Autodesk Inventor part; units mm, degrees
note: some values were not read from the file. Chosen so that the rebuilt part matches the saved one: direction of "Hole2".
(part 8 of 20)
  point P41 (-10089.727378, -10011.36586)
  point P42 (-10089.721398, -10011.390784)
  point P43 (-10089.71643, -10011.417432)
  point P44 (-10089.712492, -10011.445788)
  point P45 (-10089.709591, -10011.475889)
  point P46 (-10089.707712, -10011.507854)
  point P47 (-10089.706845, -10011.541631)
  point P48 (-10089.706982, -10011.577158)
  point P49 (-10089.708115, -10011.614374)
  point P50 (-10089.710236, -10011.653217)
  point P51 (-10091.342478, -10024.766723)
  point P52 (-10091.399992, -10024.634549)
  point P53 (-10091.454687, -10024.504325)
  point P54 (-10091.506613, -10024.375943)
  point P55 (-10091.602327, -10024.124275)
  point P56 (-10091.767293, -10025.369098)
  point P57 (-10091.726276, -10025.518742)
  point P58 (-10091.691392, -10025.662063)
  point P59 (-10091.66305, -10025.798056)
  point P60 (-10091.641632, -10025.925944)
  point P61 (-10091.627322, -10026.048439)
  point P62 (-10091.621155, -10026.162546)
  point P63 (-10091.621534, -10026.214773)
  point P64 (-10091.624365, -10026.263004)
  point P65 (-10091.629522, -10026.307033)
  point P66 (-10091.63684, -10026.346721)
  point P67 (-10091.646154, -10026.381929)
  point P68 (-10091.657297, -10026.412517)
  point P69 (-10091.685546, -10026.46165)
  point P70 (-10091.722424, -10026.49673)
  point P71 (-10091.767199, -10026.516512)
  point P72 (-10091.818874, -10026.520292)
  point P73 (-10091.875447, -10026.509788)
  point P74 (-10091.478055, -10022.118968)
  point P75 (-10091.547474, -10021.99281)
  point P76 (-10091.613916, -10021.868329)
  point P77 (-10091.67744, -10021.74542)
  point P78 (-10091.795946, -10021.503906)
  point P79 (-10091.795946, -10016.690075)
  point P80 (-10091.67744, -10016.448562)
  point P81 (-10091.613916, -10016.325653)
  point P82 (-10091.547474, -10016.201172)
  point P83 (-10091.478055, -10016.075014)
  point P84 (-10091.758883, -10022.729261)
  point P85 (-10091.707882, -10022.846777)
  point P86 (-10091.660376, -10022.960867)
  point P87 (-10091.616621, -10023.071034)
  point P88 (-10091.576871, -10023.176785)
  point P89 (-10091.541376, -10023.277639)
  point P90 (-10091.509756, -10023.375327)
  point P91 (-10091.482385, -10023.469454)
  point P92 (-10091.460347, -10023.557327)
  point P93 (-10091.444642, -10023.636373)
  point P94 (-10091.435434, -10023.705234)
  point P95 (-10091.432401, -10023.763266)
  point P96 (-10091.435236, -10023.810105)
  point P97 (-10091.443918, -10023.848166)
  point P98 (-10091.458396, -10023.877605)
  point P99 (-10091.458885, -10014.315907)
  point P100 (-10091.444621, -10014.344922)
  point P101 (-10091.435858, -10014.383099)
  point P102 (-10091.432679, -10014.430219)
  point P103 (-10091.435166, -10014.486064)
  point P104 (-10091.4434, -10014.550414)
  point P105 (-10091.457511, -10014.623566)
  point P106 (-10091.477418, -10014.705503)
  point P107 (-10091.502884, -10014.79549)
  point P108 (-10091.533671, -10014.89279)
  point P109 (-10091.56954, -10014.996669)
  point P110 (-10091.610254, -10015.106389)
  point P111 (-10091.655535, -10015.221179)
  point P112 (-10091.704831, -10015.339983)
  point P113 (-10091.602327, -10014.069706)
  point P114 (-10091.506613, -10013.818038)
  point P115 (-10091.454687, -10013.689656)
  point P116 (-10091.399992, -10013.559433)
  point P117 (-10091.342478, -10013.427258)
  point P118 (-10091.873857, -10011.683647)
  point P119 (-10091.817711, -10011.673522)
  point P120 (-10091.767253, -10011.677461)
  point P121 (-10091.723512, -10011.696704)
  point P122 (-10091.687035, -10011.731311)
  point P123 (-10091.658201, -10011.780891)
  point P124 (-10091.637389, -10011.845052)
  point P125 (-10091.624978, -10011.923403)
  point P126 (-10091.621158, -10012.016326)
  point P127 (-10091.625734, -10012.123495)
  point P128 (-10091.638501, -10012.243451)
  point P129 (-10091.659257, -10012.374739)
  point P130 (-10091.687797, -10012.5159)
  point P131 (-10091.723724, -10012.665293)
  point P132 (-10091.766103, -10012.820692)
  point P133 (-10070.533011, -10008.748999)
  point P134 (-10070.550101, -10008.752168)
  point P135 (-10070.56679, -10008.756332)
  point P136 (-10070.583016, -10008.761453)
  point P137 (-10070.598721, -10008.767492)
  point P138 (-10070.613843, -10008.774411)
  point P139 (-10070.628324, -10008.782172)
  point P140 (-10070.642102, -10008.790736)
  point P141 (-10070.655119, -10008.800064)
  point P142 (-10070.667313, -10008.81012)
  point P143 (-10070.678626, -10008.820863)
  point P144 (-10070.688996, -10008.832256)
  point P145 (-10070.698365, -10008.844261)
  point P146 (-10070.706672, -10008.856839)
  point P147 (-10070.713856, -10008.869951)
  point P148 (-10070.70671, -10009.029203)
  point P149 (-10070.699656, -10009.040668)
  point P150 (-10070.691833, -10009.051698)
  point P151 (-10070.683284, -10009.062271)
  point P152 (-10070.674052, -10009.072362)
  point P153 (-10070.664177, -10009.08195)
  point P154 (-10070.653702, -10009.091011)
  point P155 (-10070.64267, -10009.099522)
  point P156 (-10070.631122, -10009.107459)
  point P157 (-10070.6191, -10009.1148)
  point P158 (-10070.606647, -10009.121521)
  point P159 (-10070.593804, -10009.127599)
  point P160 (-10070.580613, -10009.133011)
  point P161 (-10070.567117, -10009.137734)
  point P162 (-10070.553358, -10009.141745)
  point P163 (-10070.560833, -10009.168396)
  point P164 (-10070.574308, -10009.163638)
  point P165 (-10070.587468, -10009.157958)
  point P166 (-10070.600283, -10009.151401)
  point P167 (-10070.612722, -10009.144012)
  point P168 (-10070.624756, -10009.135837)
  point P169 (-10070.636354, -10009.126921)
  point P170 (-10070.647488, -10009.11731)
  point P171 (-10070.658127, -10009.10705)
  point P172 (-10070.668242, -10009.096185)
  point P173 (-10070.677801, -10009.08476)
  point P174 (-10070.686776, -10009.072823)
  point P175 (-10070.695137, -10009.060417)
  point P176 (-10070.702854, -10009.047589)
  point P177 (-10070.709896, -10009.034384)
  point P178 (-10070.736958, -10008.893917)
  point P179 (-10070.733336, -10008.872545)
  point P180 (-10070.727426, -10008.851652)
  point P181 (-10070.719472, -10008.832002)
  point P182 (-10070.709661, -10008.813762)
  point P183 (-10070.698133, -10008.796927)
  point P184 (-10070.685027, -10008.781493)
  point P185 (-10070.670484, -10008.767455)
  point P186 (-10070.654642, -10008.754809)
  point P187 (-10070.63764, -10008.743551)
  point P188 (-10070.619619, -10008.733676)
  point P189 (-10070.600718, -10008.725181)
  point P190 (-10070.581076, -10008.71806)
  point P191 (-10070.560833, -10008.71231)
  point P192 (-10070.540128, -10008.707927)
  point P193 (-10070.388305, -10008.711852)
  point P194 (-10070.370582, -10008.717557)
  point P195 (-10070.353881, -10008.724776)
  point P196 (-10070.33824, -10008.733439)
  point P197 (-10070.323696, -10008.743478)
  point P198 (-10070.310287, -10008.754823)
  point P199 (-10070.29805, -10008.767405)
sketch "Sketch2" plane through (0, 0, 0) normal (1, 0, 0) x (0, 1, 0)
  line L0 (0, -156.78708) -> (0, 91.844197)
  line L1 (-13, 0) -> (12, 0)
  line L2 (-13, 0) -> (-13.762, 0)
  line L3 (-11, 25) -> (0, 25)
  line L4 (-11, 23.984) -> (-11, 25)
  line L5 (-8.5, 10) -> (8.5, 10)
  line L6 (8.5, 10) -> (8.5, 0)
  line L7 (8.5, 0) -> (-8.5, 0)
  line L8 (-8.5, 0) -> (-8.5, 10)
  line L9 (-12, 5) -> (12, 5)
  line L10 (12, 5) -> (12, 0)
  line L11 (12, 0) -> (-12, 0)
  line L12 (-12, 0) -> (-12, 5)
  line L13 (-7.484, 10) -> (-7.484, 0)
  line L14 (-10.984, 5) -> (-10.984, 0)
  spline S0 degree 4 poles (-11, 23.984) (-11, 20.713142) (-6.894492, 12.873224) (-7.998886, 10.368918) (-11.171855, 5.720689) (-13.556557, 3.508331) (-13.762, 1.387882) (-13.762, 0) knots 0 0 0 0 0 0.40323167 0.58584486 0.72553562 1 1 1 1 1
  spline S1 degree 4 poles (-10.457364, 23.213267) (-10.164256, 18.862838) (-2.980363, 8.550774) (-10.836637, 7.0695) (-13, 2.343966) (-13, 0) knots 0 0 0 0 0 0.54007932 1 1 1 1 1
  line L15 (-10.208157, 7.245893) -> (-13.791843, 2.754107) construction
  arc A0 (-10.476033, 6.706372) -> (-13.325291, 3.135118) centre (4.098236, -7.843675) ccw construction
  line L16 (-7.766531, 11.715278) -> (-9.233469, 8.284722) construction
  arc A1 (-9.226155, 8.730487) -> (-8.083773, 11.402041) centre (-14.334615, 12.494937) ccw construction
  line L17 (0, 23.984) -> (0, 25)
  line L18 (-13, 0) -> (-13, -15)
  line L19 (-13.762, 0) -> (-13.762, -15)
  arc A2 (-9.484, 23.984) -> (-10.457364, 23.213267) centre (-9.484, 22.984) ccw
  line L20 (-10.64831, 26.047373) -> (-10.266417, 20.379161) construction
  arc A3 (-10.271989, 25.399064) -> (-9.980462, 21.072091) centre (-3.224232, 23.700595) ccw construction
  line L21 (0, 23.984) -> (-9.484, 23.984)
  line L22 (-10.984, 23.984) -> (-11, 23.984)
  line L23 (-13.762, -15) -> (-13, -15)
  circle A4 centre (-10, 24) radius 1
  point P0 (0, 0)
  point P1 (0, 0)
  point P2 (0, 10)
  dimension "d16" = 25
  dimension "d17" = 17
  dimension "d18" = 10
  dimension "d19" = 24
  dimension "d20" = 5
  dimension "d22" = 1.016
  dimension "d23" = 1.016
  dimension "d25" = 2
  dimension "d26" = 15
  dimension "d27" = 0.762
  dimension "d28" = 13
  dimension "d91" = 11
  dimension "d92" = 2
  constraints: 46 end point, 10 parallel, 9 midpoint, 7 point on line, 5 centre point, 5 horizontal, 5 point on circle, 4 coincident, 4 perpendicular, 4 tangent, 3 vertical, 2 vertical alignment, 15 other
  measures "d16" distance between parallel lines of L1 L3
  measures "d17" distance between parallel lines of L6 L8
  measures "d18" distance between parallel lines of L7 L5
  measures "d19" distance between parallel lines of L10 L12
  measures "d20" distance between parallel lines of L11 L9
  measures "d22" distance between parallel lines of L13 L8
  measures "d23" distance between parallel lines of L14 L12
  measures "d25" diameter of A2
  measures "d26" distance of L19.end L2.end
  measures "d27" distance of L1.start L2.end
  measures "d28" distance of point (0, 0) L1.start
  measures "d91" distance of L3.end L3.start
  measures "d92" diameter of A4
revolve "Revolution1" [suppressed]
revolve "Mid Thick" add sketch "Sketch2" angle 360 about axis through (0, 0, -10) along (0, 0, 1) contours L2 L18 L23 L19
sketch "Sketch4" plane through (0, 0, 0) normal (1, 0, 0) x (0, 1, 0)
  line L0 (13.762, -15) -> (-13.762, -15)
  line L1 (0, -156.78708) -> (0, 91.844197)
  line L2 (-12, -15) -> (12, -15)
  line L3 (12, -15) -> (12, -29.976908)
  line L4 (12, -29.976908) -> (-12, -29.976908)
  line L5 (-12, -29.976908) -> (-12, -15)
  line L6 (-12, -29.976908) -> (-13.016, -29.976908)
  line L7 (-12, -25) -> (-12, -29.976908)
  line L8 (-13.762, -15) -> (-13.762, 0)
  line L9 (-13, 0) -> (-13, -15)
  spline S0 degree 4 poles (-13, -15) (-13, -16.878366) (-13, -20.635099) (-12, -24.341809) (-12, -28.098542) (-12, -29.976908) knots 0 0 0 0 0 0.5 1 1 1 1 1
  line L10 (-13.016, -29.976908) -> (-13.016, -27.488454)
  spline S1 degree 4 poles (-13.762, -15) (-13.762, -16.875595) (-13.762, -20.626785) (-13.016, -24.350123) (-13.016, -28.101313) (-13.016, -29.976908) knots 0 0 0 0 0 0.5 1 1 1 1 1
  line L11 (-13.762, -15) -> (-13, -15)
  point P0 (0, 0)
  point P1 (0, -15)
  point P2 (0, -15)
  dimension "d34" = 24
  dimension "d37" = 1.016
  constraints: 16 end point, 4 vertical, 3 parallel, 2 horizontal, 2 midpoint, 1 coincident, 1 collinear, 1 perpendicular, 1 point on line, 4 other
  measures "d34" distance between parallel lines of L3 L5
  measures "d37" distance of L4.end L6.end
revolve "Mid Tran" add sketch "Sketch4" angle 360 about axis through (0, 0, -10) along (0, 0, 1) contours S0 L6 S1 L0
sketch "Sketch5" plane through (0, 0, 0) normal (1, 0, 0) x (0, 1, 0)
  line L0 (13.016, -29.976908) -> (-13.016, -29.976908)
  line L1 (12, -29.976908) -> (-12, -29.976908)
  line L2 (0, -156.78708) -> (0, 91.844197)
  line L3 (-12, -29.976908) -> (14, -29.976908)
  line L4 (14, -29.976908) -> (14, -79.976908)
  line L5 (14, -79.976908) -> (-12, -79.976908)
  line L6 (-12, -79.976908) -> (-12, -29.976908)
  line L7 (-12, -29.976908) -> (-13.016, -29.976908)
  line L8 (-12, -79.976908) -> (-13.016, -79.976908)
  line L9 (-13.016, -79.976908) -> (-13.016, -29.976908)
  point P0 (0, 0)
  dimension "d39" = 26
  dimension "d40" = 1.016
  dimension "d41" = 50
  constraints: 14 end point, 3 parallel, 2 perpendicular, 1 horizontal
  measures "d39" distance between parallel lines of L4 L6
  measures "d40" distance of L5.end L8.end
  measures "d41" distance between parallel lines of L5 L0
revolve "Thin" add sketch "Sketch5" angle 360 about axis through (0, 0, -10) along (0, 0, 1) contours L6 L8 L9 L0
sketch "Sketch7" plane through (0, 0, -79.976908) normal (0, 0, -1) x (-1, 0, 0)
  circle A0 centre (0, 0) radius 13.016 projected
  circle A1 centre (0, 0) radius 12 projected
  circle A2 centre (0, 0) radius 13.016
  constraints: 1 centre point, 1 coincident, 1 concentric
ref_plane "Work Plane5" through (0, 0, -79.976908) normal (0, 0, 1) x (1, 0, 0)
extrude "Extrusion1" add sketch "Sketch7" along normal blind 4 contours A0 | A1
sketch "Sketch8" plane through (0, 0, -83.976908) normal (0, 0, -1) x (-1, 0, 0)
  circle A0 centre (0, 0) radius 13.016
  line L0 (7.582299, 2.074) -> (6.427599, 4.074)
  line L1 (6.427599, 4.074) -> (7.582299, 6.074)
  line L2 (7.582299, 6.074) -> (9.891701, 6.074)
  line L3 (9.891701, 6.074) -> (11.046401, 4.074)
  line L4 (11.046401, 4.074) -> (9.891701, 2.074)
  line L5 (9.891701, 2.074) -> (7.582299, 2.074)
  line L6 (0, -149.722214) -> (0, 130.927476)
  line L7 (-9.503701, 6.82) -> (-7.194299, 6.82)
  line L8 (-7.194299, 6.82) -> (-6.039599, 4.82)
  line L9 (-6.039599, 4.82) -> (-7.194299, 2.82)
  line L10 (-7.194299, 2.82) -> (-9.503701, 2.82)
  line L11 (-9.503701, 2.82) -> (-10.658401, 4.82)
  line L12 (-10.658401, 4.82) -> (-9.503701, 6.82)
  line L13 (1.154701, -7.494) -> (2.309401, -9.494)
  line L14 (2.309401, -9.494) -> (1.154701, -11.494)
  line L15 (1.154701, -11.494) -> (-1.154701, -11.494)
  line L16 (-1.154701, -11.494) -> (-2.309401, -9.494)
  line L17 (-2.309401, -9.494) -> (-1.154701, -7.494)
  line L18 (-1.154701, -7.494) -> (1.154701, -7.494)
  point P0 (8.737, 4.074)
  point P1 (-8.349, 4.82)
  point P2 (0, -9.494)
  point P3 (8.737, 4.074)
  dimension "d45" = 4.074
  dimension "d46" = 8.737
  dimension "d47" = 4.82
  dimension "d48" = 8.349
  dimension "d49" = 9.494
  dimension "d51" = 4
  dimension "d52" = 4
  dimension "d53" = 4
  constraints: 36 end point, 1 coincident, 1 other
  measures "d45" vertical distance of point (8.737, 4.074) A0.centre
  measures "d46" horizontal distance of point (8.737, 4.074) A0.centre
  measures "d47" vertical distance of point (-8.349, 4.82) A0.centre
  measures "d48" horizontal distance of A0.centre point (-8.349, 4.82)
  measures "d49" distance of point (0, -9.494) A0.centre
  measures "d51" distance between parallel lines of L0 L3
  measures "d52" distance between parallel lines of L7 L10
  measures "d53" distance between parallel lines of L13 L16
hole "Hole1" at (-8.737, 4.074, -83.976908) at (8.349, 4.82, -83.976908) at (0, -9.494, -83.976908) at (-8.737, 4.074, -83.976908) direction (0, 0, 1) diameter 1.778 depth 4 clearance for "Flat Head Machine Screw (82)" size "#0" standard "Ansi Unified Screw Threads"
sketch "Sketch9" plane through (0, 0, 0) normal (1, 0, 0) x (0, 1, 0)
  line L0 (-13.016, -83.976908) -> (-13.016, -29.976908)
  line L1 (13.016, -83.976908) -> (-13.016, -83.976908)
  line L2 (0, -156.78708) -> (0, 91.844197)
  line L3 (-8, -83.976908) -> (0, -83.976908)
  line L4 (0, -83.976908) -> (0, -103.976908)
  line L5 (0, -103.976908) -> (-5, -103.976908)
  spline S0 degree 3 poles (-13.016, -83.976908) (-13.016, -91.416878) (-13.016, -98.856848) (-5, -103.976908) knots 0 0 0 0 1 1 1 1
  line L6 (-13.016, -83.976908) -> (-8, -83.976908)
  point P0 (0, 0)
  point P1 (-4, -83.976908)
  dimension "d68" = 20
  dimension "d102" = 5
  constraints: 8 end point, 2 midpoint, 1 coincident, 1 horizontal, 1 horizontal alignment, 1 parallel, 1 perpendicular, 1 vertical, 2 other
  measures "d68" distance between parallel lines of L5 L3
  measures "d102" distance of L4.end L5.end
revolve "Revolution6" add sketch "Sketch9" angle 360 about axis through (0, 0, -10) along (0, 0, 1)
ref_plane "Work Plane6" through (0, 0, -82.476908) normal (0, 0, 1) x (1, 0, 0)
sketch "Sketch11" plane through (0, 0, -82.476908) normal (0, 0, 1) x (1, 0, 0)
  circle A0 centre (-8.737, 4.074) radius 0.889
  circle A1 centre (8.349, 4.82) radius 0.889
  circle A2 centre (0, -9.494) radius 0.889
  line L0 (-9.891701, 2.074) -> (-7.582299, 2.074)
  line L1 (-11.046401, 4.074) -> (-9.891701, 2.074)
  line L2 (-7.582299, 2.074) -> (-6.427599, 4.074)
  line L3 (-9.891701, 6.074) -> (-11.046401, 4.074)
  line L4 (-7.582299, 6.074) -> (-9.891701, 6.074)
  line L5 (-6.427599, 4.074) -> (-7.582299, 6.074)
  line L6 (1.154701, -7.494) -> (-1.154701, -7.494)
  line L7 (2.309401, -9.494) -> (1.154701, -7.494)
  line L8 (1.154701, -11.494) -> (2.309401, -9.494)
  line L9 (-1.154701, -11.494) -> (1.154701, -11.494)
  line L10 (-2.309401, -9.494) -> (-1.154701, -11.494)
  line L11 (-1.154701, -7.494) -> (-2.309401, -9.494)
  line L12 (7.194299, 6.82) -> (6.039599, 4.82)
  line L13 (9.503701, 6.82) -> (7.194299, 6.82)
  line L14 (10.658401, 4.82) -> (9.503701, 6.82)
  line L15 (9.503701, 2.82) -> (10.658401, 4.82)
  line L16 (7.194299, 2.82) -> (9.503701, 2.82)
  line L17 (6.039599, 4.82) -> (7.194299, 2.82)
  point P0 (0, 0)
extrude "Extrusion3" cut sketch "Sketch11" against normal through all contours A0 | A1 | A2 | L1 L3 L4 L5 L2 L0 | L7 L8 L9 L10 L11 L6 | L13 L14 L15 L16 L17 L12
ref_plane "Work Plane7" through (0, 0, -79.976908) normal (0, 0, 1) x (1, 0, 0)
hole "Hole2" at (0, 0, -103.976908) direction (0, 0, 1) diameter 10 depth 24
sketch "Sketch12" plane through (0, 0, 0) normal (1, 0, 0) x (0, 1, 0)
  spline S0 degree 3 poles (67.040686, -110.340683) (67.181711, -110.754373) (67.468131, -111.594574) (67.844542, -112.900649) (68.165475, -114.276843) (68.403591, -115.689425) (68.553461, -117.090576) (68.628909, -118.438876) (68.654169, -119.741368) (68.654209, -120.596035) (68.654229, -121.018326) knots 0 0 0 0 0.13110718 0.26627767 0.40758133 0.55482273 0.69573025 0.83010398 0.95981582 1.08650249 1.08650249 1.08650249 1.08650249
  spline S1 degree 3 poles (65.040686, -106.036195) (65.040686, -106.035984) (65.040686, -106.035137) (65.040686, -106.033234) (65.040686, -106.030066) (65.040686, -106.025636) (65.040686, -106.019951) (65.040686, -106.013017) (65.040686, -106.004838) (65.040686, -105.99542) (65.040686, -105.984769) (65.040686, -105.972891) (65.040686, -105.959801) (65.040686, -105.945517) (65.040686, -105.930056) (65.040686, -105.913432) (65.040686, -105.895658) (65.040686, -105.883426) (65.040686, -105.877121) knots 0 0 0 0 0.00398745 0.01595749 0.03589091 0.06374884 0.09949715 0.14310174 0.1945285 0.2537433 0.32071204 0.39540061 0.47774624 0.56757484 0.66479437 0.76932497 0.8810868 1 1 1 1
  spline S2 degree 3 poles (65.040686, -105.877121) (65.194176, -106.260743) (65.498781, -107.022054) (66.173784, -108.506895) (66.69415, -109.607645) (67.040686, -110.340683) knots 0 0 0 0 0.25334256 0.50276707 1 1 1 1
  spline S3 degree 3 poles (83.354686, -109.977444) (83.205067, -110.403955) (82.900857, -111.271152) (82.494774, -112.619657) (82.145236, -114.043985) (81.88387, -115.507795) (81.718837, -116.959462) (81.635693, -118.354075) (81.607874, -119.699651) (81.607833, -120.582214) (81.607812, -121.018326) knots 0 0 0 0 0.13558682 0.27568002 0.42231514 0.57532331 0.7214304 0.86036495 0.99429907 1.12513191 1.12513191 1.12513191 1.12513191
  line L0 (81.354686, -105.464425) -> (81.354686, -121.018326)
  line L1 (81.607812, -121.018326) -> (81.354686, -121.018326)
  line L2 (81.354686, -121.018326) -> (79.354686, -121.018326)
  spline S4 degree 3 poles (79.354686, -121.018326) (79.354686, -120.136015) (79.354686, -118.791551) (79.354686, -116.963337) (79.354686, -115.515321) (79.354686, -114.054436) (79.354686, -112.629922) (79.354686, -111.279853) (79.354686, -110.404808) (79.354686, -109.977141) knots 0 0 0 0 0.26469338 0.4033392 0.54846434 0.69909791 0.84160494 0.97581833 1.10411856 1.10411856 1.10411856 1.10411856
  spline S5 degree 3 poles (79.354686, -109.977141) (79.707447, -109.240902) (80.237826, -108.133962) (80.818531, -106.821015) (81.133082, -106.053241) (81.280528, -105.661469) (81.354686, -105.464425) knots 0 0 0 0 0.49596798 0.74569065 0.8720938 1 1 1 1
  spline S6 degree 3 poles (81.354686, -105.464425) (81.436258, -105.489435) (81.598942, -105.539315) (81.848975, -105.589935) (82.101098, -105.62152) (82.354754, -105.631933) (82.608329, -105.621551) (82.860555, -105.589985) (83.110519, -105.539404) (83.273215, -105.489542) (83.354686, -105.464572) knots 0 0 0 0 0.12572609 0.25074567 0.37552827 0.50000542 0.62458391 0.74924522 0.87443269 1 1 1 1
  spline S7 degree 3 poles (83.354686, -105.464572) (83.354686, -105.853913) (83.354686, -106.619619) (83.354686, -108.123909) (83.354686, -109.238859) (83.354686, -109.977444) knots 0 0 0 0 0.25882001 0.5090148 1 1 1 1
  line L3 (67.040686, -94.518326) -> (67.040686, -110.340683)
  line L4 (67.040686, -94.518326) -> (69.040686, -94.518326)
  line L5 (69.040686, -94.518326) -> (69.040686, -121.018326)
  line L6 (65.040686, -94.518326) -> (65.040686, -105.877121)
  line L7 (65.040686, -94.518326) -> (67.040686, -94.518326)
  line L8 (79.354686, -94.518326) -> (79.354686, -109.977141)
  line L9 (79.354686, -94.518326) -> (81.354686, -94.518326)
  line L10 (81.354686, -94.518326) -> (81.354686, -105.464425)
  line L11 (81.354686, -94.518326) -> (83.354686, -94.518326)
  line L12 (83.354686, -94.518326) -> (83.354686, -105.464572)
  line L13 (78.608686, -94.518326) -> (78.608686, -121.018326)
  line L14 (78.608686, -94.518326) -> (79.354686, -94.518326)
  line L15 (80.608686, -94.518326) -> (80.608686, -121.018326)
  line L16 (82.608686, -94.518326) -> (82.608686, -110.485254)
  spline S8 degree 3 poles (80.987443, -121.018326) (80.987462, -120.601747) (80.987501, -119.758823) (81.01289, -118.474335) (81.088746, -117.144746) (81.239448, -115.762632) (81.478869, -114.368665) (81.801344, -113.01032) (82.179342, -111.721556) (82.467066, -110.89305) (82.608686, -110.485254) knots 0 0 0 0 0.12497306 0.25287553 0.38537145 0.52436553 0.66974205 0.80937847 0.9429718 1.07246485 1.07246485 1.07246485 1.07246485
  spline S9 degree 3 poles (82.608686, -105.721075) (82.52253, -105.726584) (82.350319, -105.737597) (82.091245, -105.726689) (81.83373, -105.695808) (81.578795, -105.643474) (81.327626, -105.571102) (81.081461, -105.479205) (80.840427, -105.370299) (80.686114, -105.284214) (80.608686, -105.24102) knots 0 0 0 0 0.12386032 0.2475762 0.37158497 0.495852 0.6207493 0.74643209 0.87276965 1 1 1 1
  spline S10 degree 3 poles (80.608686, -105.24102) (80.536619, -105.426978) (80.393173, -105.797117) (80.085372, -106.522873) (79.67593, -107.411332) (79.152243, -108.458702) (78.790042, -109.149046) (78.608686, -109.494703) knots 0 0 0 0 0.12719878 0.25318248 0.50275428 0.75102731 1 1 1 1
  line L17 (88.534686, -92.018326) -> (64.534686, -92.018326)
  line L18 (86.018686, 21.942582) -> (67.050686, 21.942582)
  line L19 (86.505368, 21.557215) -> (66.564004, 21.557215)
  spline S11 degree 3 poles (65.550686, 2.958582) (65.696442, 3.15771) (65.990398, 3.559307) (66.63789, 4.332671) (67.316977, 5.091944) (67.96316, 5.888495) (68.33248, 6.417332) (68.593779, 6.863991) (68.769836, 7.213831) (68.926202, 7.578332) (69.008957, 7.831116) (69.050686, 7.958582) knots 0 0 0 0 0.07401284 0.14926686 0.30244691 0.37959616 0.45685507 0.49566205 0.53474567 0.5742877 0.61450742 0.61450742 0.61450742 0.61450742
  spline S12 degree 3 poles (87.518686, 2.958582) (87.37293, 3.15771) (87.078974, 3.559307) (86.431482, 4.332671) (85.752395, 5.091944) (85.106213, 5.888495) (84.736892, 6.417332) (84.475593, 6.863991) (84.299536, 7.213831) (84.14317, 7.578332) (84.060415, 7.831116) (84.018686, 7.958582) knots 0 0 0 0 0.07401284 0.14926686 0.30244691 0.37959616 0.45685507 0.49566205 0.53474567 0.5742877 0.61450742 0.61450742 0.61450742 0.61450742
  spline S13 degree 3 poles (64.034686, -2.041418) (64.037832, -1.818607) (64.04412, -1.373262) (64.103581, -0.708699) (64.209137, -0.052784) (64.368677, 0.589154) (64.583246, 1.213523) (64.853982, 1.817393) (65.174985, 2.402355) (65.424915, 2.772377) (65.550686, 2.958582) knots 0 0 0 0 0.06683217 0.13358148 0.19996019 0.26595386 0.33177154 0.39774949 0.46426825 0.53165054 0.53165054 0.53165054 0.53165054
  spline S14 degree 3 poles (89.034686, -2.041418) (89.03154, -1.818607) (89.025252, -1.373262) (88.965791, -0.708699) (88.860235, -0.052784) (88.700695, 0.589154) (88.486126, 1.213523) (88.215391, 1.817393) (87.894387, 2.402355) (87.644457, 2.772377) (87.518686, 2.958582) knots 0 0 0 0 0.06683217 0.13358148 0.19996019 0.26595386 0.33177154 0.39774949 0.46426825 0.53165054 0.53165054 0.53165054 0.53165054
  arc A0 (86.505368, 21.557215) -> (86.018686, 21.942582) centre (86.018686, 21.442582) ccw
  arc A1 (67.050686, 21.942582) -> (66.564004, 21.557215) centre (67.050686, 21.442582) ccw
  spline S15 degree 3 poles (69.050686, 7.958582) (69.104819, 8.159433) (69.215638, 8.570605) (69.299992, 9.222432) (69.32743, 9.914929) (69.289863, 10.650133) (69.193528, 11.426673) (69.041848, 12.243358) (68.83889, 13.097233) (68.505279, 14.303469) (68.009186, 15.861647) (67.384973, 17.757913) (66.925594, 19.360458) (66.657385, 20.629559) (66.594637, 21.25291) (66.564004, 21.557215) knots 0 0 0 0 0.06234657 0.1276327 0.1966407 0.27004939 0.34820305 0.43123424 0.51911498 0.61142292 0.80662861 1.00959387 1.21035176 1.30648489 1.39817641 1.39817641 1.39817641 1.39817641
  spline S16 degree 3 poles (84.018686, 7.958582) (83.964553, 8.159433) (83.853734, 8.570605) (83.769381, 9.222432) (83.741942, 9.914929) (83.77951, 10.650133) (83.875844, 11.426673) (84.027524, 12.243358) (84.230482, 13.097233) (84.564093, 14.303469) (85.060187, 15.861647) (85.684399, 17.757913) (86.143778, 19.360458) (86.411987, 20.629559) (86.474736, 21.25291) (86.505368, 21.557215) knots 0 0 0 0 0.06234657 0.1276327 0.1966407 0.27004939 0.34820305 0.43123424 0.51911498 0.61142292 0.80662861 1.00959387 1.21035176 1.30648489 1.39817641 1.39817641 1.39817641 1.39817641
  line L20 (87.534686, 22.958582) -> (65.534686, 22.958582)
  spline S17 degree 3 poles (68.034686, 7.958582) (67.934145, 7.742514) (67.730909, 7.305746) (67.355975, 6.67586) (66.947859, 6.044593) (66.506986, 5.411639) (66.037254, 4.782076) (65.376039, 3.96496) (64.87044, 3.36019) (64.534686, 2.958582) knots 0 0 0 0 0.07145122 0.1444341 0.21963753 0.29697342 0.37578786 0.45523025 0.61227239 0.61227239 0.61227239 0.61227239
  spline S18 degree 3 poles (85.034686, 7.958582) (85.135227, 7.742514) (85.338463, 7.305746) (85.713398, 6.67586) (86.121513, 6.044593) (86.562387, 5.411639) (87.032119, 4.782076) (87.693333, 3.96496) (88.198933, 3.36019) (88.534686, 2.958582) knots 0 0 0 0 0.07145122 0.1444341 0.21963753 0.29697342 0.37578786 0.45523025 0.61227239 0.61227239 0.61227239 0.61227239
  spline S19 degree 3 poles (64.534686, 2.958582) (64.391139, 2.773942) (64.177438, 2.499066) (63.921801, 2.115667) (63.74796, 1.825722) (63.592502, 1.530213) (63.456028, 1.22896) (63.339682, 0.921485) (63.243369, 0.607961) (63.166118, 0.288773) (63.087618, -0.145209) (63.032036, -0.699119) (63.015615, -1.369168) (63.017663, -1.817428) (63.018686, -2.041418) knots 0 0 0 0 0.07013118 0.1044054 0.13817293 0.17150982 0.2045203 0.23732848 0.27006639 0.30285264 0.33579 0.40230943 0.46959172 0.53678969 0.53678969 0.53678969 0.53678969
  spline S20 degree 3 poles (88.534686, 2.958582) (88.678233, 2.773942) (88.891934, 2.499066) (89.147571, 2.115667) (89.321413, 1.825722) (89.476871, 1.530213) (89.613344, 1.22896) (89.72969, 0.921485) (89.826003, 0.607961) (89.903254, 0.288773) (89.981754, -0.145209) (90.037337, -0.699119) (90.053758, -1.369168) (90.05171, -1.817428) (90.050686, -2.041418) knots 0 0 0 0 0.07013118 0.1044054 0.13817293 0.17150982 0.2045203 0.23732848 0.27006639 0.30285264 0.33579 0.40230943 0.46959172 0.53678969 0.53678969 0.53678969 0.53678969
  spline S21 degree 3 poles (65.534686, 21.942582) (65.55153, 21.625542) (65.586982, 20.958222) (65.799755, 19.936612) (66.079405, 18.863014) (66.530055, 17.400852) (67.022889, 15.959413) (67.492662, 14.551628) (67.805168, 13.564577) (68.06678, 12.638691) (68.268386, 11.780568) (68.404564, 10.992675) (68.468083, 10.273449) (68.458204, 9.618811) (68.379378, 9.021526) (68.239024, 8.4702) (68.102158, 8.127516) (68.034686, 7.958582) knots 0 0 0 0 0.09512154 0.200216 0.31218274 0.42803367 0.65906444 0.76919754 0.87325746 0.96964043 1.05776849 1.13759246 1.20931346 1.27406394 1.33359113 1.38967504 1.44420495 1.44420495 1.44420495 1.44420495
  spline S22 degree 3 poles (87.534686, 21.942582) (87.517843, 21.625542) (87.48239, 20.958222) (87.269617, 19.936612) (86.989967, 18.863014) (86.539318, 17.400852) (86.046483, 15.959413) (85.57671, 14.551628) (85.264205, 13.564577) (85.002592, 12.638691) (84.800986, 11.780568) (84.664809, 10.992675) (84.60129, 10.273449) (84.611168, 9.618811) (84.689994, 9.021526) (84.830348, 8.4702) (84.967214, 8.127516) (85.034686, 7.958582) knots 0 0 0 0 0.09512154 0.200216 0.31218274 0.42803367 0.65906444 0.76919754 0.87325746 0.96964043 1.05776849 1.13759246 1.20931346 1.27406394 1.33359113 1.38967504 1.44420495 1.44420495 1.44420495 1.44420495
  line L21 (65.534686, 21.942582) -> (65.534686, 22.958582)
  line L22 (87.534686, 21.942582) -> (87.534686, 22.958582)
  line L23 (84.534686, -121.018326) -> (81.607812, -121.018326)
  line L24 (79.354686, -121.018326) -> (68.654229, -121.018326)
  spline S23 degree 3 poles (63.518686, -96.018326) (63.519479, -96.870586) (63.520667, -98.146747) (63.621473, -99.842752) (63.759935, -101.104322) (63.970024, -102.355857) (64.256379, -103.595658) (64.611615, -104.825029) (64.897293, -105.631431) (65.040686, -106.036195) knots 0 0 0 0 0.25561003 0.38274706 0.50949551 0.6361782 0.76322409 0.89103186 1.01983443 1.01983443 1.01983443 1.01983443
  spline S24 degree 3 poles (89.550686, -96.018326) (89.546142, -97.088345) (89.539339, -98.690067) (89.355839, -100.815549) (89.097312, -102.390762) (88.720342, -103.947002) (88.078134, -106.008624) (87.042686, -108.518326) (86.007238, -111.028028) (85.36503, -113.08965) (84.98806, -114.645891) (84.729533, -116.221103) (84.546034, -118.346586) (84.539231, -119.948307) (84.534686, -121.018326) knots 0 0 0 0 0.32084871 0.48028147 0.63946219 0.79924314 0.96029185 1.28673686 1.61318187 1.77423059 1.93401153 2.09319225 2.25262502 2.57347372 2.57347372 2.57347372 2.57347372
  line L25 (81.534686, -92.018326) -> (81.534686, -121.018326)
  line L26 (71.534686, -92.018326) -> (71.534686, -121.018326)
  line L27 (81.497686, -92.018326) -> (81.497686, -94.518326)
  line L28 (79.719686, -92.018326) -> (79.719686, -94.518326)
  line L29 (82.243686, -92.018326) -> (82.243686, -94.518326)
  line L30 (80.465686, -92.018326) -> (80.465686, -94.518326)
  line L31 (67.929686, -92.018326) -> (67.929686, -94.518326)
  line L32 (66.151686, -92.018326) -> (66.151686, -94.518326)
  line L33 (64.534686, -92.018326) -> (64.534686, -32.018326)
  line L34 (88.534686, -92.018326) -> (88.534686, -32.018326)
  line L35 (63.518686, -96.018326) -> (63.518686, -32.018326)
  line L36 (89.550686, -96.018326) -> (89.550686, -32.018326)
  spline S25 degree 3 poles (64.534686, -32.018326) (64.534349, -31.809534) (64.533674, -31.392358) (64.495675, -30.767061) (64.408772, -30.145712) (64.284686, -29.529872) (64.1606, -28.914033) (64.073697, -28.292684) (64.035698, -27.667387) (64.035024, -27.250211) (64.034686, -27.041418) knots 0 0 0 0 0.0626312 0.12513986 0.18776052 0.25067229 0.31358405 0.37620471 0.43871337 0.50134457 0.50134457 0.50134457 0.50134457
  spline S26 degree 3 poles (88.534686, -32.018326) (88.535024, -31.809534) (88.535698, -31.392358) (88.573697, -30.767061) (88.6606, -30.145712) (88.784686, -29.529872) (88.908772, -28.914033) (88.995675, -28.292684) (89.033674, -27.667387) (89.034349, -27.250211) (89.034686, -27.041418) knots 0 0 0 0 0.0626312 0.12513986 0.18776052 0.25067229 0.31358405 0.37620471 0.43871337 0.50134457 0.50134457 0.50134457 0.50134457
  spline S27 degree 3 poles (63.018686, -27.041418) (63.019024, -27.250211) (63.019698, -27.667387) (63.057697, -28.292684) (63.1446, -28.914033) (63.268686, -29.529872) (63.392772, -30.145712) (63.479675, -30.767061) (63.517674, -31.392358) (63.518349, -31.809534) (63.518686, -32.018326) knots 0 0 0 0 0.0626312 0.12513986 0.18776052 0.25067229 0.31358405 0.37620471 0.43871337 0.50134457 0.50134457 0.50134457 0.50134457
  spline S28 degree 3 poles (90.050686, -27.041418) (90.050349, -27.250211) (90.049674, -27.667387) (90.011675, -28.292684) (89.924772, -28.914033) (89.800686, -29.529872) (89.6766, -30.145712) (89.589697, -30.767061) (89.551698, -31.392358) (89.551024, -31.809534) (89.550686, -32.018326) knots 0 0 0 0 0.0626312 0.12513986 0.18776052 0.25067229 0.31358405 0.37620471 0.43871337 0.50134457 0.50134457 0.50134457 0.50134457
  line L37 (64.034686, -27.041418) -> (64.034686, -2.041418)
  line L38 (89.034686, -27.041418) -> (89.034686, -2.041418)
  line L39 (63.018686, -27.041418) -> (63.018686, -2.041418)
  line L40 (90.050686, -27.041418) -> (90.050686, -2.041418)
  line L41 (-90.466621, -35.917041) -> (-90.442087, -35.912003)
  ellipse E0 centre (-90.343602, -35.894235) end of major axis (-89.559894, -35.733604) minor radius 0.002388 (-90.187105, -35.859771) -> (-90.442087, -35.912003) ccw
  ellipse E1 centre (-90.343602, -35.894235) end of major axis (-89.559894, -35.733604) minor radius 0.002388 (-89.559894, -35.733604) -> (-90.01196, -35.824053) ccw
  line L42 (-89.559756, -35.73428) -> (-89.559894, -35.733604)
  ellipse E2 centre (-103.65948, -35.894235) end of major axis (-104.443188, -35.733604) minor radius 0.002388 (-103.992479, -35.823777) -> (-104.443188, -35.733604) ccw
  line L43 (-102.646483, -36.098913) -> (-102.414014, -36.146449)
  line L44 (-104.443326, -35.73428) -> (-104.443188, -35.733604)
  ellipse E3 centre (-90.875964, -36.03792) end of major axis (-90.117864, -35.782412) minor radius 0.00228 (-90.80754, -36.012462) -> (-90.958968, -36.063503) ccw
  ellipse E4 centre (-90.875964, -36.03792) end of major axis (-90.117864, -35.782412) minor radius 0.00228 (-90.689307, -35.972678) -> (-90.801699, -36.010495) ccw
  ellipse E5 centre (-90.875964, -36.03792) end of major axis (-90.117864, -35.782412) minor radius 0.00228 (-90.117864, -35.782412) -> (-90.289361, -35.838691) ccw
  line L45 (-90.11513, -35.790524) -> (-90.117864, -35.782412)
  line L46 (-92.674489, -35.892021) -> (-94.327933, -30.986199)
  ellipse E6 centre (-88.233607, -36.951348) end of major axis (-89.011017, -37.140116) minor radius 0.136933 (-88.528399, -36.890417) -> (-88.545422, -36.895726) ccw
  line L47 (-88.816146, -36.96257) -> (-88.62556, -36.912263)
  ellipse E7 centre (-88.00113, -37.90877) end of major axis (-88.487012, -38.02675) minor radius 0.085583 (-88.121508, -37.851839) -> (-88.268041, -38.045128) ccw
  ellipse E8 centre (-106.692039, -35.867548) end of major axis (-107.491785, -35.8877) minor radius 0.133925 (-107.04331, -35.755799) -> (-107.491785, -35.8877) ccw
  line L48 (-106.719125, -35.734323) -> (-105.145649, -35.686856)
  line L49 (-105.145649, -35.686856) -> (-105.140676, -35.88423)
  ellipse E9 centre (-106.642372, -37.838699) end of major axis (-107.442118, -37.85885) minor radius 0.133925 (-106.370354, -37.706058) -> (-106.669458, -37.705473) ccw
  line L50 (-105.145649, -35.686856) -> (-105.155563, -35.29341)
  line L51 (-105.172568, -34.618497) -> (-105.1969, -33.652856)
  ellipse E10 centre (-107.037224, -22.168053) end of major axis (-109.126561, -22.220698) minor radius 0.349879 (-107.891271, -21.869557) -> (-108.146045, -21.898574) ccw
  ellipse E11 centre (-107.014874, -23.055071) end of major axis (-109.104211, -23.107715) minor radius 0.349879 (-107.877588, -22.757441) -> (-108.11313, -22.784232) ccw
  ellipse E12 centre (-107.014874, -23.055071) end of major axis (-108.514398, -23.092854) minor radius 0.251109 (-106.221205, -22.822514) -> (-108.470628, -23.150977) ccw
  ellipse E13 centre (-106.642372, -37.838699) end of major axis (-107.142214, -37.851293) minor radius 0.083703 (-106.716086, -37.757691) -> (-106.890842, -37.917435) ccw
  ellipse E14 centre (-104.240205, -35.814279) end of major axis (-105.038162, -35.757144) minor radius 0.002347 (-104.354333, -35.803779) -> (-105.038162, -35.757144) ccw
  line L52 (-104.354333, -35.803779) -> (-104.295665, -35.807955)
  line L53 (-104.059089, -35.824793) -> (-102.799639, -35.914435)
  line L54 (-102.799639, -35.914435) -> (-102.814933, -36.128042)
  line L55 (-105.039107, -35.770331) -> (-105.038162, -35.757144)
  line L56 (-102.799639, -35.914435) -> (-102.680421, -34.24943)
  line L57 (-90.880231, -35.479301) -> (-90.812485, -35.821466)
  line L58 (-91.848425, -36.30283) -> (-90.375139, -36.031417)
  ellipse E15 centre (-90.307773, -35.920377) end of major axis (-89.523007, -35.765) minor radius 0.096422 (-90.375139, -36.031417) -> (-89.66586, -35.73864) ccw
  line L59 (-89.66586, -35.73864) -> (-90.18766, -35.747597)
  line L60 (-89.521474, -35.772742) -> (-89.523007, -35.765)
  line L61 (-88.366054, -35.597257) -> (-88.355181, -35.701091)
  line L62 (-88.871729, -35.904988) -> (-87.996085, -35.808354)
  ellipse E16 centre (-87.889599, -35.831286) end of major axis (-87.093949, -35.747968) minor radius 0.034185 (-87.129232, -35.741687) -> (-87.996085, -35.808354) ccw
  ellipse E17 centre (-89.335927, -22.019504) end of major axis (-87.257293, -21.801836) minor radius 0.089309 (-87.399609, -21.784456) -> (-87.900814, -21.804539) ccw
  ellipse E18 centre (-89.24228, -22.913792) end of major axis (-87.163646, -22.696124) minor radius 0.089309 (-87.308637, -22.678729) -> (-87.376049, -22.679181) ccw
  ellipse E19 centre (-87.681494, -37.818593) end of major axis (-88.178775, -37.870667) minor radius 0.021366 (-88.057958, -37.843906) -> (-88.155364, -37.861609) ccw
  ellipse E20 centre (-87.681494, -37.818593) end of major axis (-87.184213, -37.766519) minor radius 0.021366 (-87.224132, -37.762354) -> (-87.493652, -37.779068) ccw
  ellipse E21 centre (-100.301556, -37.154438) end of major axis (-99.595388, -37.300356) minor radius 0.431228 (-101.009802, -37.10384) -> (-100.993099, -37.166903) ccw
  line L63 (-104.697671, -35.209096) -> (-104.756287, -35.768848)
  ellipse E22 centre (-106.113483, -35.831286) end of major axis (-105.317834, -35.914604) minor radius 0.034185 (-106.14405, -35.793745) -> (-106.846869, -35.7413) ccw
  line L64 (-106.14405, -35.793745) -> (-105.130983, -35.897952)
  line L65 (-104.561105, -35.784903) -> (-104.501911, -35.219625)
  ellipse E23 centre (-104.667155, -22.019504) end of major axis (-106.745789, -21.801836) minor radius 0.089309 (-106.102268, -21.804539) -> (-106.603473, -21.784456) ccw
  ellipse E24 centre (-104.760802, -22.913792) end of major axis (-106.839436, -22.696124) minor radius 0.089309 (-106.627033, -22.679181) -> (-106.694445, -22.678729) ccw
  ellipse E25 centre (-104.760802, -22.913792) end of major axis (-106.252645, -22.757571) minor radius 0.064098 (-106.212405, -22.747195) -> (-106.215765, -22.775958) ccw
  ellipse E26 centre (-106.321588, -37.818593) end of major axis (-105.824307, -37.870667) minor radius 0.021366 (-105.855185, -37.874796) -> (-105.945124, -37.843906) ccw
  ellipse E27 centre (-106.321588, -37.818593) end of major axis (-106.818869, -37.766519) minor radius 0.021366 (-106.50943, -37.779068) -> (-106.787599, -37.777382) ccw
  line L66 (-101.826025, -33.176696) -> (-102.425721, -36.205579)
  line L67 (-104.130028, -35.752776) -> (-104.207956, -35.745992)
  ellipse E28 centre (-103.695309, -35.920377) end of major axis (-104.480075, -35.765) minor radius 0.096422 (-104.207956, -35.745992) -> (-103.820309, -35.993013) ccw
  line L68 (-103.820309, -35.993013) -> (-102.294711, -36.321317)
  line L69 (-102.294711, -36.321317) -> (-102.303894, -36.367694)
  line L70 (-104.481608, -35.772742) -> (-104.480075, -35.765)
  line L71 (-102.350104, -36.286019) -> (-102.294711, -36.321317)
  line L72 (-102.294711, -36.321317) -> (-101.67558, -33.194274)
  line L73 (-90.012444, -35.829859) -> (-89.844365, -35.817773)
  ellipse E29 centre (-89.762877, -35.814279) end of major axis (-88.96492, -35.757144) minor radius 0.002347 (-88.96492, -35.757144) -> (-89.844365, -35.817773) ccw
  line L74 (-88.963976, -35.770331) -> (-88.96492, -35.757144)
  line L75 (-91.608122, -33.121203) -> (-91.608901, -33.110315)
  line L76 (-87.734507, -35.527633) -> (-87.739358, -35.720134)
  line L77 (-88.95241, -35.73049) -> (-87.421684, -35.732161)
  ellipse E30 centre (-87.311043, -35.867548) end of major axis (-86.511297, -35.8877) minor radius 0.133925 (-86.511297, -35.8877) -> (-87.421684, -35.732161) ccw
  ellipse E31 centre (-86.965858, -22.168053) end of major axis (-89.055195, -22.115408) minor radius 0.349879 (-85.857037, -21.898574) -> (-86.111811, -21.869557) ccw
  ellipse E32 centre (-86.988208, -23.055071) end of major axis (-89.077545, -23.002426) minor radius 0.349879 (-85.889952, -22.784232) -> (-86.125494, -22.757441) ccw
  ellipse E33 centre (-86.988208, -23.055071) end of major axis (-85.488684, -23.092854) minor radius 0.251109 (-85.552513, -23.162744) -> (-87.781877, -22.822514) ccw
  ellipse E34 centre (-87.335876, -36.853124) end of major axis (-88.135623, -36.832973) minor radius 0.133925 (-87.446517, -36.717736) -> (-87.466538, -36.717758) ccw
  ellipse E35 centre (-87.36071, -37.838699) end of major axis (-87.860551, -37.826104) minor radius 0.083703 (-87.11224, -37.917435) -> (-87.089062, -37.915636) ccw
  ellipse E36 centre (-87.36071, -37.838699) end of major axis (-86.860869, -37.851293) minor radius 0.083703 (-87.035815, -37.783027) -> (-87.286996, -37.757691) ccw
  line L78 (-105.300401, -36.919594) -> (-105.186074, -36.946173)
  ellipse E37 centre (-105.769475, -36.951348) end of major axis (-106.546885, -36.762581) minor radius 0.136933 (-105.45766, -36.895726) -> (-105.476237, -36.889936) ccw
  ellipse E38 centre (-106.001952, -37.90877) end of major axis (-105.516071, -38.02675) minor radius 0.085583 (-105.735041, -38.045128) -> (-105.881574, -37.851839) ccw
  ellipse E39 centre (-103.127118, -36.03792) end of major axis (-103.885218, -35.782412) minor radius 0.00228 (-103.715025, -35.838256) -> (-103.885218, -35.782412) ccw
  line L79 (-101.907552, -36.988982) -> (-102.062587, -37.448979)
  line L80 (-103.887952, -35.790524) -> (-103.885218, -35.782412)
  line L81 (-101.002593, -34.303939) -> (-99.76883, -30.643326)
  line L82 (-101.823309, -37.323227) -> (-102.062587, -37.448979)
  line L83 (-102.062587, -37.448979) -> (-102.085947, -37.441338)
  line L84 (-102.385663, -37.340223) -> (-102.062587, -37.448979)
  line L85 (-90.647195, -35.958269) -> (-90.491351, -35.923747)
  ellipse E40 centre (-90.41167, -35.908741) end of major axis (-89.630547, -35.735978) minor radius 0.002568 (-90.363003, -35.895352) -> (-90.491351, -35.923747) ccw
  ellipse E41 centre (-90.41167, -35.908741) end of major axis (-89.630547, -35.735978) minor radius 0.002568 (-90.246715, -35.869687) -> (-90.359974, -35.894683) ccw
  ellipse E42 centre (-90.41167, -35.908741) end of major axis (-89.630547, -35.735978) minor radius 0.002568 (-89.630547, -35.735978) -> (-90.047847, -35.825947) ccw
  line L86 (-89.630098, -35.738006) -> (-89.630547, -35.735978)
  ellipse E43 centre (-87.682192, -37.955636) end of major axis (-86.887089, -37.867253) minor radius 0.263102 (-88.36863, -38.157355) -> (-88.222424, -38.203335) ccw
  ellipse E44 centre (-87.682192, -37.955636) end of major axis (-86.887089, -37.867253) minor radius 0.263102 (-87.12084, -38.087535) -> (-86.956317, -37.992095) ccw
  ellipse E45 centre (-106.32089, -37.955636) end of major axis (-107.115993, -37.867253) minor radius 0.263102 (-106.850174, -37.705716) -> (-107.001172, -37.751093) ccw
  ellipse E46 centre (-106.32089, -37.955636) end of major axis (-107.115993, -37.867253) minor radius 0.263102 (-107.031465, -37.766275) -> (-107.040417, -37.771491) ccw
  ellipse E47 centre (-106.32089, -37.955636) end of major axis (-107.115993, -37.867253) minor radius 0.263102 (-107.10701, -37.918597) -> (-106.882242, -38.087535) ccw
  ellipse E48 centre (-106.32089, -37.955636) end of major axis (-105.525788, -38.044019) minor radius 0.263102 (-105.780658, -38.203335) -> (-105.634452, -38.157355) ccw
  line L87 (-92.595907, -36.698352) -> (-92.476971, -36.652156)
  ellipse E49 centre (-91.066352, -36.106911) end of major axis (-90.320547, -35.817472) minor radius 0.002457 (-90.944638, -36.057075) -> (-90.96114, -36.063471) ccw
  ellipse E50 centre (-91.066352, -36.106911) end of major axis (-90.320547, -35.817472) minor radius 0.002457 (-90.850305, -36.020544) -> (-90.898721, -36.039288) ccw
  ellipse E51 centre (-91.066352, -36.106911) end of major axis (-90.320547, -35.817472) minor radius 0.002457 (-90.320547, -35.817472) -> (-90.392082, -35.844111) ccw
  line L88 (-92.23411, -37.630604) -> (-92.595907, -36.698352)
  ellipse E52 centre (-90.342759, -37.971415) end of major axis (-91.088564, -38.260854) minor radius 0.002457 (-90.64361, -38.085759) -> (-90.633261, -38.086582) ccw
  line L89 (-91.088564, -38.260854) -> (-91.450361, -37.328602)
  line L90 (-90.314652, -35.832662) -> (-90.320547, -35.817472)
  line L91 (-92.595907, -36.698352) -> (-94.528229, -31.719281)
  line L92 (-91.449479, -37.330874) -> (-92.23411, -37.630604)
  line L93 (-92.23411, -37.630604) -> (-92.584487, -37.445278)
  ellipse E53 centre (-92.256707, -37.320066) end of major axis (-93.13149, -36.935364) minor radius 0.25544 (-93.12843, -37.008649) -> (-92.584487, -37.445278) ccw
  line L94 (-93.12843, -37.008649) -> (-94.629248, -33.141448)
  ellipse E54 centre (-90.704556, -37.039163) end of major axis (-91.450361, -37.328602) minor radius 0.002457 (-91.303967, -37.270217) -> (-91.450361, -37.328602) ccw
  line L95 (-92.23411, -37.630604) -> (-91.308663, -37.271155)
  ellipse E55 centre (-90.342759, -37.971415) end of major axis (-90.808887, -38.152314) minor radius 0.001536 (-90.641196, -38.085968) -> (-90.63575, -38.086401) ccw
  ellipse E56 centre (-88.372874, -36.995775) end of major axis (-89.141558, -37.217419) minor radius 0.14613 (-88.582568, -36.90793) -> (-88.814488, -36.994129) ccw
  line L96 (-88.81539, -36.97697) -> (-88.590296, -36.908632)
  ellipse E57 centre (-88.10048, -37.940463) end of major axis (-88.580907, -38.078991) minor radius 0.091331 (-88.123754, -37.852122) -> (-88.259637, -38.074276) ccw
  ellipse E58 centre (-88.10048, -37.940463) end of major axis (-88.869163, -38.162107) minor radius 0.14613 (-88.427677, -37.893938) -> (-88.36863, -38.157355) ccw
  line L97 (-88.869163, -38.162107) -> (-88.980258, -37.776821)
  line L98 (-96.395902, -34.951561) -> (-96.424259, -34.494843)
  line L99 (-101.481122, -37.376572) -> (-101.403848, -37.512643)
  line L100 (-101.403848, -37.512643) -> (-100.927038, -37.405753)
  ellipse E59 centre (-99.649245, -37.924209) end of major axis (-100.422508, -38.129305) minor radius 0.142054 (-100.422508, -38.129305) -> (-100.004857, -38.145751) ccw
  line L101 (-100.422508, -38.129305) -> (-100.597624, -37.469073)
  line L102 (-106.201839, -35.707777) -> (-106.210602, -35.53446)
  line L103 (-105.454516, -35.610182) -> (-105.451459, -35.670651)
  ellipse E60 centre (-106.80357, -35.880709) end of major axis (-107.602549, -35.921103) minor radius 0.142983 (-107.08625, -35.760642) -> (-107.602549, -35.921103) ccw
  line L104 (-106.805974, -35.737668) -> (-105.23306, -35.659845)
  line L105 (-105.23306, -35.659845) -> (-105.231564, -35.689448)
  ellipse E61 centre (-106.704211, -37.845996) end of major axis (-107.503191, -37.88639) minor radius 0.142983 (-107.024001, -37.730452) -> (-107.046765, -37.992095) ccw
  ellipse E62 centre (-106.704211, -37.845996) end of major axis (-107.503191, -37.88639) minor radius 0.142983 (-106.433427, -37.698056) -> (-106.706615, -37.702955) ccw
  line L106 (-107.503191, -37.88639) -> (-107.602549, -35.921103)
  line L107 (-105.23306, -35.659845) -> (-105.234833, -35.624783)
  line L108 (-105.286537, -34.602089) -> (-105.328044, -33.781091)
  line L109 (-106.420238, -35.718583) -> (-106.430885, -35.507997)
  ellipse E63 centre (-107.494113, -22.221966) end of major axis (-109.581447, -22.327495) minor radius 0.373543 (-108.146045, -21.898574) -> (-109.581447, -22.327495) ccw
  ellipse E64 centre (-107.449401, -23.106345) end of major axis (-109.536735, -23.211874) minor radius 0.373543 (-108.11313, -22.784232) -> (-109.084094, -23.418928) ccw
  line L110 (-109.581447, -22.327495) -> (-109.536735, -23.211874)
  ellipse E65 centre (-107.449401, -23.106345) end of major axis (-108.947488, -23.182084) minor radius 0.268093 (-106.229194, -22.890892) -> (-108.791739, -23.291232) ccw
  ellipse E66 centre (-106.704211, -37.845996) end of major axis (-107.203573, -37.871242) minor radius 0.089364 (-106.719759, -37.757325) -> (-106.889795, -37.938145) ccw
  line L111 (-103.566564, -35.788711) -> (-103.543957, -35.358559)
  line L112 (-102.928195, -34.221654) -> (-102.938407, -34.415957)
  line L113 (-102.991669, -35.429377) -> (-103.015078, -35.874784)
  ellipse E67 centre (-104.325204, -35.809007) end of major axis (-105.124102, -35.76702) minor radius 0.002573 (-104.416161, -35.801666) -> (-105.124102, -35.76702) ccw
  line L114 (-104.416161, -35.801666) -> (-102.853693, -35.883206)
  line L115 (-102.853693, -35.883206) -> (-102.855127, -35.910486)